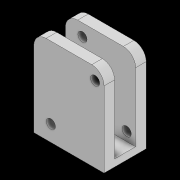
# Autodesk Inventor part: Sujetador_radar
Saved by Autodesk Inventor 2022 (Build 260153000, 153)
## iProperties
Created: 2021-10-20
Part Number: Sujetador_radar
Material: Genérico
Document SubType Name: Modeling
Designer: Julio R
Density: 1 g/cm^3
Appearance: Valor por defecto
Author: Julio R
Autodesk Inventor part; units mm, degrees
ref_plane "YZ Plane" through (0, 0, 0) normal (1, 0, 0) x (0, 1, 0)
ref_plane "XZ Plane" through (0, 0, 0) normal (0, 1, 0) x (-1, 0, 0)
ref_plane "XY Plane" through (0, 0, 0) normal (0, 0, 1) x (1, 0, 0)
sketch "Boceto1" plane through (0, 0, 0) normal (0, 1, 0) x (-1, 0, 0)
  circle A0 centre (0, 0) radius 1.7
  line L0 (-10, -3) -> (10, -3)
  line L1 (10, -3) -> (10, 3)
  line L2 (10, 3) -> (-10, 3)
  line L3 (-10, 3) -> (-10, -3)
  line L4 (-10, -3) -> (10, 3) construction
  line L5 (10, -3) -> (-10, 3) construction
  line L6 (10, 3) -> (-10, 3)
  line L7 (-10, 3) -> (-10, 6)
  line L8 (-10, 6) -> (10, 6)
  line L9 (10, 6) -> (10, 3)
  line L10 (10, -3) -> (-10, -3)
  line L11 (-10, -3) -> (-10, -6)
  line L12 (-10, -6) -> (10, -6)
  line L13 (10, -6) -> (10, -3)
  dimension "d0" = 3.4
  dimension "d1" = 20
  dimension "d2" = 6
  dimension "d3" = 3
  dimension "d4" = 3
  constraints: 28 end point, 6 parallel, 3 horizontal, 3 perpendicular, 2 midpoint, 1 centre point, 1 coincident, 1 point on line
  measures "d0" diameter of A0
  measures "d1" distance of L2.end L1.end
  measures "d2" distance of L1.end L0.end
  measures "d3" distance of L6.end L7.end
  measures "d4" distance of L11.end L10.end
extrude "Extrusión1" add sketch "Boceto1" against normal blind 2 contours L3 L2 L1 L0
extrude "Extrusión2" add sketch "Boceto1" along normal blind 23 contours L0 L13 L12 L11 | L7 L8 L9 L2
sketch "Boceto2" plane through (-10, 0, 6) normal (0, 0, 1) x (1, 0, 0)
  line L0 (0, 0) -> (20, 0) projected
  line L1 (20, 0) -> (20, 23) projected
  line L2 (0, 23) -> (20, 23) projected
  line L3 (0, 0) -> (0, 23) projected
  circle A0 centre (17.46, 2.54) radius 1.2989
  circle A1 centre (17.46, 19.54) radius 1.2989
  circle A2 centre (4.86, 2.54) radius 1.2989
  circle A3 centre (4.86, 19.54) radius 1.2989
  point P0 (10, 0)
  dimension "d9" = 2.54
  dimension "d10" = 2.54
  dimension "d13" = 17
  dimension "d16" = 12.6
  constraints: 4 centre point, 1 horizontal, 1 vertical, 6 other
  measures "d9" distance from line of L0 A0.centre
  measures "d10" distance from line of L1 A0.centre
  measures "d13" distance of A0.centre A1.centre
  measures "d16" distance of A0.centre A2.centre
extrude "Extrusión3" cut sketch "Boceto2" against normal up to surface (3 mm away) contours A1 | A2
extrude "Extrusión4" add sketch "Boceto1" against normal blind 2 contours L0 L13 L12 L11 | L7 L8 L9 L2
extrude "Extrusión5" cut sketch "Boceto2" along normal up to surface (3 mm away) from surface at -12 contours A0 | A3
fillet "Empalme1" radius 3.5 4 edges at (-10, 23, 4.5) (-10, 23, -4.5) (10, 23, -4.5) (10, 23, 4.5)
